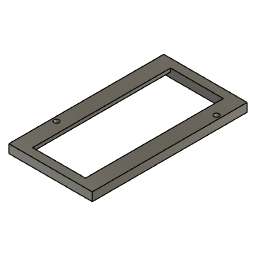
CarteProtect v2 (Autodesk Fusion 360 design; units mm, degrees)
Autodesk Fusion 360 part; units mm, degrees
sketch "Esquisse1" plane through (0, 0, 0) normal (0, 0, 1) x (1, 0, 0)
  line L0 (0, 0) -> (-36, 0)
  line L1 (-36, 0) -> (-36, 80)
  line L2 (-36, 80) -> (0, 80)
  line L3 (0, 80) -> (0, 0)
  line L4 (-36.5, 80.5) -> (0.5, 80.5)
  line L5 (0.5, 80.5) -> (0.5, -0.5)
  line L6 (0.5, -0.5) -> (-36.5, -0.5)
  line L7 (-36.5, -0.5) -> (-36.5, 80.5)
  line L8 (-38.5, 82.5) -> (2.5, 82.5)
  line L9 (2.5, 82.5) -> (2.5, -2.5)
  line L10 (2.5, -2.5) -> (-38.5, -2.5)
  line L11 (-38.5, -2.5) -> (-38.5, 82.5)
  circle A0 centre (4, 70.04) radius 1.5
  circle A1 centre (4, 70.04) radius 3
  circle A2 centre (-40, 19.95) radius 1.5
  circle A3 centre (-40, 19.95) radius 3
  line L12 (-42.5, 85.5) -> (6.5, 85.5)
  line L13 (6.5, 85.5) -> (6.5, -5.5)
  line L14 (6.5, -5.5) -> (-42.5, -5.5)
  line L15 (-42.5, -5.5) -> (-42.5, 85.5)
  dimension "d1" = 36
  dimension "d2" = 80
  dimension "d3" = 0.5
  dimension "d4" = 0.5
  dimension "d5" = 0.5
  dimension "d6" = 0.5
  dimension "d7" = 2
  dimension "d8" = 2
  dimension "d9" = 2
  dimension "d10" = 2
  dimension "d11" = 3
  dimension "d12" = 9.96
  dimension "d13" = 4
  dimension "d14" = 6
  dimension "d15" = 3
  dimension "d16" = 4
  dimension "d17" = 6
  dimension "d18" = 19.95
  dimension "d19" = 3
  dimension "d20" = 4
  dimension "d21" = 4
  dimension "d22" = 3
  constraint horizontal L0
  constraint vertical L1
  constraint horizontal L2
  constraint vertical L3
  constraint coincident L0.start L3.end
  constraint horizontal L4
  constraint vertical L5
  constraint horizontal L6
  constraint vertical L7
  constraint horizontal L8
  constraint vertical L9
  constraint horizontal L10
  constraint vertical L11
  constraint concentric A0 A1
  constraint concentric A2 A3
  constraint horizontal L12
  constraint vertical L13
  constraint horizontal L14
  constraint vertical L15
  measures "d1" distance of L1.end L2.end
  measures "d2" distance of L0.end L1.end
  measures "d3" distance of L1 L7
  measures "d4" distance of L3 L5
  measures "d5" distance of L2 L4
  measures "d6" distance of L0 L6
  measures "d7" distance of L4 L8
  measures "d8" distance of L7 L11
  measures "d9" distance of L5 L9
  measures "d10" distance of L6 L10
  measures "d11" diameter of A0
  measures "d12" distance of L2 A0.centre
  measures "d13" distance of L3 A0.centre
  measures "d14" diameter of A1
  measures "d15" diameter of A2
  measures "d16" distance of L1 A2.centre
  measures "d17" diameter of A3
  measures "d18" distance of L0 A2.centre
  measures "d19" distance of L8 L12
  measures "d20" distance of L11 L15
  measures "d21" distance of L9 L13
  measures "d22" distance of L10 L14
extrude "Extrusion1" add sketch "Esquisse1" along normal blind 3 contours L8 L9 L11 A1 A3 L12 L13 L15 | L8 L9 L10 L11 A1 A3 | L11 A3 | L11 A3 L15 | L9 A1 L13 | L9 A1 | L9 L10 L11 A1 A3 L13 L14 L15
sketch "Esquisse2" plane through (0, 0, 3) normal (0, 0, 1) x (-1, 0, 0)
  circle A0 centre (40, -19.95) radius 1.5
  circle A1 centre (-4, -70.04) radius 1.5
  line L0 (-0.5, 0.5) -> (36.5, 0.5)
  line L1 (36.5, 0.5) -> (36.5, -80.5)
  line L2 (36.5, -80.5) -> (-0.5, -80.5)
  line L3 (-0.5, -80.5) -> (-0.5, 0.5)
  line L4 (42.5, 5.5) -> (-6.5, 5.5)
  line L5 (-6.5, 5.5) -> (-6.5, -85.5)
  line L6 (-6.5, -85.5) -> (42.5, -85.5)
  line L7 (42.5, -85.5) -> (42.5, 5.5)
  line L8 (36.5, -80.5) -> (33.5, -80.5)
  line L9 (33.5, -80.5) -> (33.5, 0.5)
  line L10 (33.5, 0.5) -> (36.5, 0.5)
  line L11 (36.5, 0.5) -> (36.5, -80.5)
  line L12 (-0.5, -80.5) -> (2.5, -80.5)
  line L13 (2.5, -80.5) -> (2.5, 0.5)
  line L14 (2.5, 0.5) -> (-0.5, 0.5)
  line L15 (-0.5, 0.5) -> (-0.5, -80.5)
  dimension "d25" = 3
  dimension "d26" = 3
  constraint horizontal L8
  constraint vertical L9
  constraint horizontal L10
  constraint vertical L11
  constraint coincident L0 L9.end
  constraint coincident L1.end L2.start
  constraint horizontal L12
  constraint vertical L13
  constraint horizontal L14
  constraint vertical L15
  constraint coincident L0 L13.end
  constraint coincident L2.end L3.start
  measures "d25" distance of L9 L11
  measures "d26" distance of L13 L15
extrude "Extrusion2" add sketch "Esquisse2" along normal blind 2 contours L0 L2 L3 L12 L13 L14 L15 | L0 L1 L2 L8 L9 L10 L11 | L4 L5 L6 L7
